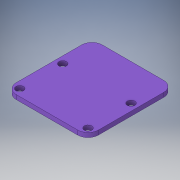
# Autodesk Inventor part: PiCameraWithMechanicalLayout
Saved by Autodesk Inventor 2019.2 (Build 232265000, 265)
## iProperties
Created: 2018-12-18
Part Number: PiCameraWithMechanicalLayout
Material: LCP Plastic
Document SubType Name: Modeling
Designer: steele
Density: 1.626 g/cm^3
Appearance: Violet
Author: steele
Autodesk Inventor part; units mm, degrees
ref_plane "YZ Plane" through (0, 0, 0) normal (1, 0, 0) x (0, 1, 0)
ref_plane "XZ Plane" through (0, 0, 0) normal (0, 1, 0) x (-1, 0, 0)
ref_plane "XY Plane" through (0, 0, 0) normal (0, 0, 1) x (1, 0, 0)
sketch "Sketch1" plane through (0, 0, 0) normal (0, 1, 0) x (-1, 0, 0)
  line L0 (11.931, 12.5) -> (-11.931, 12.5)
  line L1 (-11.931, 12.5) -> (-11.931, -12.5)
  line L2 (-11.931, -12.5) -> (11.931, -12.5)
  line L3 (11.931, -12.5) -> (11.931, 12.5)
  line L4 (11.931, 12.5) -> (-11.931, -12.5) construction
  line L5 (-11.931, 12.5) -> (11.931, -12.5) construction
  point P0 (0, 0)
  point P1 (-29, 11.5)
  point P2 (-29, -11.5)
  dimension "d0" = 23.862
  dimension "d1" = 25
  constraints: 12 end point, 2 midpoint, 2 parallel, 1 horizontal, 1 perpendicular
  measures "d0" distance of L0.start L0.end
  measures "d1" distance of L2.end L0.start
extrude "Extrusion1" add sketch "Sketch1" against normal blind 1.27
fillet "Fillet1" radius 3 4 edges at (-11.931, -0.635, 12.5) (11.931, -0.635, 12.5) (11.931, -0.635, -12.5) (-11.931, -0.635, -12.5)
sketch "Sketch3" plane through (0, 0, 0) normal (0, 1, 0) x (1, 0, 0)
  line L0 (9.931, -10.5) -> (-9.931, -10.5) construction
  line L1 (-9.931, -10.5) -> (-9.931, 2) construction
  line L2 (-9.931, 2) -> (9.931, 2) construction
  line L3 (9.931, 2) -> (9.931, -10.5) construction
  line L4 (-8.931, -12.5) -> (8.931, -12.5) projected
  line L5 (11.931, -9.5) -> (11.931, 9.5) projected
  line L6 (-11.931, 9.5) -> (-11.931, -9.5) projected
  point P0 (0, 0)
  dimension "d16" = 2
  dimension "d17" = 2
  dimension "d18" = 2
  dimension "d19" = 14.5
  constraints: 8 end point, 4 coincident, 2 parallel, 1 horizontal, 1 perpendicular
  measures "d16" distance between parallel lines of L0 L4
  measures "d17" distance between parallel lines of L5 L3
  measures "d18" distance between parallel lines of L1 L6
  measures "d19" distance between parallel lines of L2 L4
hole "Hole2" at (9.931, 0, 10.5) at (9.931, 0, -2) at (-9.931, 0, -2) at (-9.931, 0, 10.5) direction (0, -1, 0) diameter 2.2 end through all
equation "\"d0\" = PiCameraLength"
equation "\"d1\" = PiCameraWidth"
equation "\"d4\" = PiZeroWHeight"
equation "\"PiZeroWHeight\" = 1.27"
equation "\"PiCameraWidth\" = 25"
equation "\"PiCameraLength\" = 23.862"
body "Solid1"
